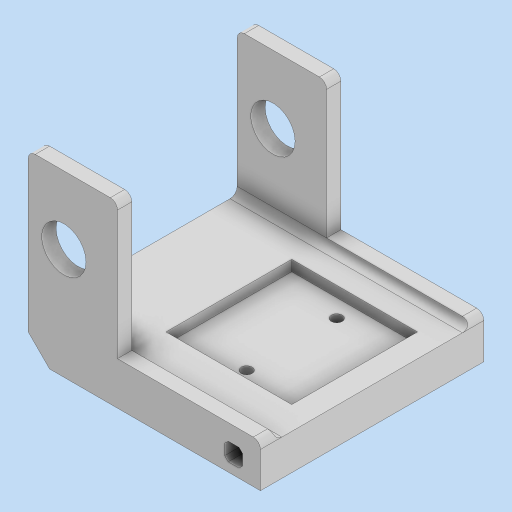
# Autodesk Inventor part: base_engrane
Saved by Autodesk Inventor 2024 (Build 280153000, 153)
## iProperties
Created: 2024-09-04
Part Number: base_engrane
Material: Generic
Document SubType Name: Modeling
Designer: MxMon
Density: 1 g/cm^3
Appearance: Default
Author: MxMon
Autodesk Inventor part; units mm, degrees
ref_plane "YZ Plane" through (0, 0, 0) normal (1, 0, 0) x (0, 1, 0)
ref_plane "XZ Plane" through (0, 0, 0) normal (0, 1, 0) x (-1, 0, 0)
ref_plane "XY Plane" through (0, 0, 0) normal (0, 0, 1) x (1, 0, 0)
sketch "Sketch1" plane through (0, 0, 0) normal (0, 1, 0) x (-1, 0, 0)
  line L0 (17.5, 31.25) -> (-17.5, 31.25)
  line L1 (-17.5, 31.25) -> (-17.5, -31.25)
  line L2 (-17.5, -31.25) -> (17.5, -31.25)
  line L3 (17.5, -31.25) -> (17.5, 31.25)
  line L4 (17.5, 31.25) -> (-17.5, -31.25) construction
  line L5 (-17.5, 31.25) -> (17.5, -31.25) construction
  point P0 (0, 0)
  dimension "d0" = 35
  dimension "d1" = 62.5
  constraints: 12 end point, 2 midpoint, 2 parallel, 1 horizontal, 1 perpendicular
  measures "d0" distance of L2.end L1.end
  measures "d1" distance of L1.end L0.end
extrude "Extrusion1" add sketch "Sketch1" along normal blind 50
sketch "Sketch2" plane through (0, 50, 0) normal (0, 1, 0) x (1, 0, 0)
  line L0 (17.5, -31.25) -> (17.5, 31.25) projected
  line L1 (-17.5, -27.25) -> (17.5, -27.25)
  line L2 (17.5, -27.25) -> (17.5, 27.25)
  line L3 (17.5, 27.25) -> (-17.5, 27.25)
  line L4 (-17.5, 27.25) -> (-17.5, -27.25)
  line L5 (-17.5, -27.25) -> (17.5, 27.25) construction
  line L6 (17.5, -27.25) -> (-17.5, 27.25) construction
  line L7 (-17.5, -31.25) -> (17.5, -31.25) projected
  point P0 (0, 0)
  point P1 (17.5, -27.25)
  dimension "d4" = 4
  constraints: 12 end point, 2 midpoint, 2 parallel, 1 horizontal, 1 perpendicular, 1 point on line
  measures "d4" distance between parallel lines of L7 L1
extrude "Extrusion2" cut sketch "Sketch2" against normal blind 40
sketch "Sketch3" plane through (-17.5, 0, 31.25) normal (0, 0, 1) x (1, 0, 0)
  circle A0 centre (10, 31) radius 6.2
  line L0 (35, 10) -> (0, 10) projected
  line L1 (35, 10) -> (35, 50) projected
  line L2 (0, 0) -> (0, 50) projected
  point P0 (17.5, 0)
  point P1 (35, 30)
  dimension "d7" = 12.4
  dimension "d15" = 21
  dimension "d38" = 10
  constraints: 1 centre point, 1 midpoint
  measures "d7" diameter of A0
  measures "d15" vertical distance of L0.start A0.centre
  measures "d38" distance from line of L2 A0.centre
extrude "Extrusion3" cut sketch "Sketch3" against normal blind 8
sketch "Sketch4" plane through (17.5, 0, -31.25) normal (0, 0, -1) x (-1, 0, 0)
  circle A0 centre (25, 31) radius 6.2 projected
  point P0 (17.5, 0)
extrude "Extrusion4" cut sketch "Sketch4" against normal blind 8
fillet "Fillet1" radius 2 2 edges at (0, 10, 27.25) (0, 10, -27.25)
sketch "Sketch5" plane through (17.5, 0, 31.25) normal (1, 0, 0) x (0, 0, -1)
  line L0 (4, 12) -> (4, 50) projected
  line L1 (0, 50) -> (4, 50) projected
  line L2 (0, 0) -> (0, 50) projected
  arc A0 (4, 12) -> (6, 10) centre (6, 12) ccw projected
  line L3 (0, 0) -> (62.5, 0) projected
  line L4 (56.5, 10) -> (6, 10) projected
  arc A1 (56.5, 10) -> (58.5, 12) centre (56.5, 12) ccw projected
  line L5 (58.5, 50) -> (58.5, 12) projected
  line L6 (62.5, 0) -> (62.5, 50) projected
  line L7 (58.5, 50) -> (62.5, 50) projected
  point P0 (31.25, 0)
extrude "Extrusion5" add sketch "Sketch5" along normal blind 30
sketch "Sketch6" plane through (0, 10, 0) normal (0, 1, 0) x (1, 0, 0)
  line L0 (5.8, 19.2) -> (41, 19.2)
  line L1 (41, 19.2) -> (41, -16)
  line L2 (41, -16) -> (5.8, -16)
  line L3 (5.8, -16) -> (5.8, 19.2)
  line L4 (5.8, 19.2) -> (41, -16) construction
  line L5 (41, 19.2) -> (5.8, -16) construction
  line L6 (-17.5, -25.25) -> (-17.5, 25.25) projected
  point P0 (0, 0)
  point P1 (23.4, 1.6)
  point P2 (-17.5, 0)
  point P3 (41, 1.6)
  point P4 (-17.5, 0)
  dimension "d16" = 35.2
  dimension "d17" = 35.2
  dimension "d84" = 1.6
  dimension "d108" = 58.5
  constraints: 12 end point, 5 midpoint, 2 parallel, 1 horizontal, 1 perpendicular
  measures "d16" distance of L1.end L2.end
  measures "d17" distance of L0.end L1.end
  measures "d84" vertical distance of point (0, 0) point (23.4, 1.6)
  measures "d108" horizontal distance of point (-17.5, 0) point (41, 1.6)
extrude "Extrusion6" cut sketch "Sketch6" against normal blind 3
sketch "Sketch10" plane through (0, 0, 0) normal (0, -1, 0) x (1, 0, 0)
  line L0 (41, 16) -> (5.8, 16) projected
  line L1 (41, -19.2) -> (41, 16) projected
  line L2 (5.8, -19.2) -> (41, -19.2) projected
  line L3 (5.8, 16) -> (5.8, -19.2) projected
  point P0 (0, 0)
  point P1 (23.4, -14.2)
  point P2 (23.4, -19.2)
  dimension "d37" = 5
  constraints: 1 midpoint, 1 vertical alignment
  measures "d37" distance from line of point (23.4, -14.2) L2
hole "Hole1" at (23.4, 0, -14.2) direction (0, 1, 0) diameter 3.1 end through all countersink diameter 4 countersink angle 90
ref_plane "Work Plane1" through (22.5, 0, -31.25) normal (-1, 0, 0) x (0, 0, 1)
fillet "Fillet4" radius 2 4 edges at (-17.5, 50, -29.25) (47.5, 50, -29.25) (47.5, 50, 29.25) (-17.5, 50, 29.25)
sketch "Sketch16" plane through (47.5, 0, -31.25) normal (0, 0, -1) x (-1, 0, 0)
  line L0 (63, 50) -> (2, 50) projected
  arc A0 (2, 50) -> (0, 48) centre (2, 48) ccw projected
  line L1 (0, 0) -> (0, 48) projected
  line L2 (0, 12) -> (65, 12) projected
  line L3 (40, 50) -> (40, 12)
  point P0 (47.5, 0)
  dimension "d93" = 40
  constraints: 2 end point, 2 point on line
  measures "d93" distance between parallel lines of L1 L3
extrude "Extrusion14" cut sketch "Sketch16" against normal blind 4
fillet "Fillet5" radius 2 1 edges at (7.5, 50, -29.25)
sketch "Sketch17" plane through (-17.5, 0, 31.25) normal (0, 0, 1) x (1, 0, 0)
  line L0 (2, 50) -> (63, 50) projected
  line L1 (65, 48) -> (65, 0) projected
  arc A0 (65, 48) -> (63, 50) centre (63, 48) ccw projected
  line L2 (0, 12) -> (65, 12) projected
  line L3 (25, 50) -> (25, 12)
  point P0 (17.5, 0)
  dimension "d88" = 40
  constraints: 2 end point, 2 point on line, 1 vertical
  measures "d88" distance between parallel lines of L1 L3
extrude "Extrusion15" cut sketch "Sketch17" against normal blind 4
fillet "Fillet6" radius 2 2 edges at (47.5, 12, 29.25) (47.5, 12, -29.25)
fillet "Fillet7" radius 2 1 edges at (7.5, 50, 29.25)
ref_plane "Work Plane2" through (41, 10, -1.6) normal (0, 0, -1) x (-1, 0, 0)
mirror "Mirror5" about plane through (41, 10, -1.6) normal (0, 0, -1) of "Hole1"
chamfer "Chamfer1" distance 6 angle 45 1 edges at (-17.5, 0, 0)
sketch "Sketch18" plane through (5.5, 50, -31.25) normal (0, 0, -1) x (-1, 0, 0)
  line L0 (-37, -42.5) -> (-32, -42.5)
  line L1 (-32, -42.5) -> (-32, -47.5)
  line L2 (-32, -47.5) -> (-37, -47.5)
  line L3 (-37, -47.5) -> (-37, -42.5)
  line L4 (-42, -50) -> (-42, -40) projected
  point P0 (5.5, -50)
  point P1 (-42, -45)
  point P2 (-37, -45)
  point P3 (-42, -45)
  dimension "d98" = 5
  dimension "d99" = 5
  dimension "d100" = 5
  constraints: 8 end point, 3 midpoint, 2 parallel, 1 horizontal, 1 horizontal alignment, 1 perpendicular
  measures "d98" distance of L0.end L1.end
  measures "d99" distance of L1.end L2.end
  measures "d100" distance from line of point (-42, -45) L3
extrude "Extrusion16" cut sketch "Sketch18" against normal blind 10
chamfer "Chamfer2" distance 1 angle 45 4 edges at (42.5, 7.5, -26.25) (37.5, 7.5, -26.25) (37.5, 2.5, -26.25) (42.5, 2.5, -26.25)
sketch "Sketch19" plane through (7.5, 12, 31.25) normal (0, 0, 1) x (1, 0, 0)
  line L0 (34, -4.5) -> (31, -4.5) projected
  line L1 (30, -5.5) -> (31, -4.5) projected
  line L2 (30, -5.5) -> (30, -8.5) projected
  line L3 (31, -9.5) -> (30, -8.5) projected
  line L4 (31, -9.5) -> (34, -9.5) projected
  line L5 (35, -8.5) -> (34, -9.5) projected
  line L6 (35, -8.5) -> (35, -5.5) projected
  line L7 (34, -4.5) -> (35, -5.5) projected
  point P0 (-7.5, -12)
extrude "Extrusion17" cut sketch "Sketch19" against normal blind 10
body "Solid1"
